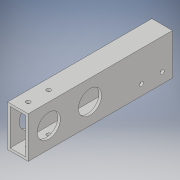
# Autodesk Inventor part: Top Roller Wheel Mount
Saved by Autodesk Inventor 2018 (Build 220112000, 112)
## iProperties
Created: 2020-02-21
Part Number: Top Roller Wheel Mount
Material: Generic
Document SubType Name: Modeling
Designer: T3500STATIC
Density: 1 g/cm^3
Appearance: Default
Author: T3500STATIC
Autodesk Inventor part; units mm, degrees
ref_plane "YZ Plane" through (0, 0, 0) normal (1, 0, 0) x (0, 1, 0)
ref_plane "XZ Plane" through (0, 0, 0) normal (0, 1, 0) x (-1, 0, 0)
ref_plane "XY Plane" through (0, 0, 0) normal (0, 0, 1) x (1, 0, 0)
sketch "Sketch1" plane through (0, 0, 0) normal (1, 0, 0) x (0, 1, 0)
  line L0 (0, 0) -> (50.8, 0)
  line L1 (50.8, 0) -> (50.8, -177.8)
  line L2 (50.8, -177.8) -> (0, -177.8)
  line L3 (0, -177.8) -> (0, 0)
  dimension "d0" = 50.8
  dimension "d1" = 177.8
  constraints: 8 end point, 2 parallel, 1 horizontal, 1 perpendicular
  measures "d0" distance of L1.end L2.end
  measures "d1" distance of L0.end L1.end
extrude "Extrusion1" add sketch "Sketch1" along normal blind 25.4
shell "Shell1" thickness 3.175 removed faces 2 at (8.4667, 16.9333, 0) at (8.4667, 33.8667, -177.8)
sketch "Sketch2" plane through (25.4, 0, 0) normal (1, 0, 0) x (0, 0, -1)
  line L0 (0, 3.175) -> (0, 47.625) construction
  line L1 (0, 25.4) -> (177.8, 25.4) construction
  line L2 (177.8, 3.175) -> (177.8, 47.625) construction
  line L3 (0, 25.4) -> (25.4, 25.4) construction
  circle A0 centre (25.4, 25.4) radius 14.2875
  line L4 (25.4, 25.4) -> (76.2, 25.4) construction
  circle A1 centre (76.2, 25.4) radius 14.2875
  circle A2 centre (25.4, 25.4) radius 19.05 construction
  circle A3 centre (76.2, 25.4) radius 19.05 construction
  line L5 (177.8, 50.8) -> (0, 50.8) construction
  line L6 (0, 50.8) -> (12.7, 50.8) construction
  line L7 (12.7, 50.8) -> (12.7, 38.1) construction
  line L8 (12.7, 38.1) -> (0, 38.1) construction
  line L9 (0, 38.1) -> (0, 50.8) construction
  line L10 (0, 0) -> (12.7, 0) construction
  line L11 (12.7, 0) -> (12.7, 12.7) construction
  line L12 (12.7, 12.7) -> (0, 12.7) construction
  line L13 (0, 12.7) -> (0, 0) construction
  line L14 (177.8, 50.8) -> (165.1, 50.8) construction
  line L15 (165.1, 50.8) -> (165.1, 38.1) construction
  line L16 (165.1, 38.1) -> (177.8, 38.1) construction
  line L17 (177.8, 38.1) -> (177.8, 50.8) construction
  line L18 (177.8, 0) -> (165.1, 0) construction
  line L19 (165.1, 0) -> (165.1, 12.7) construction
  line L20 (165.1, 12.7) -> (177.8, 12.7) construction
  line L21 (177.8, 12.7) -> (177.8, 0) construction
  line L22 (177.8, 50.8) -> (139.7, 50.8) construction
  line L23 (139.7, 50.8) -> (139.7, 38.1) construction
  line L24 (139.7, 38.1) -> (177.8, 38.1) construction
  line L25 (177.8, 38.1) -> (177.8, 50.8) construction
  line L26 (177.8, 0) -> (139.7, 0) construction
  line L27 (139.7, 0) -> (139.7, 12.7) construction
  line L28 (139.7, 12.7) -> (177.8, 12.7) construction
  line L29 (177.8, 12.7) -> (177.8, 0) construction
  circle A4 centre (165.1, 12.7) radius 2.5797
  circle A5 centre (139.7, 12.7) radius 2.5797
  dimension "d5" = 25.4
  dimension "d6" = 28.575
  dimension "d7" = 50.8
  dimension "d8" = 28.575
  dimension "d9" = 38.1
  dimension "d10" = 38.1
  dimension "d11" = 12.7
  dimension "d12" = 12.7
  dimension "d13" = 12.7
  dimension "d14" = 12.7
  dimension "d15" = 12.7
  dimension "d16" = 12.7
  dimension "d17" = 12.7
  dimension "d18" = 12.7
  dimension "d19" = 38.1
  dimension "d20" = 38.1
  dimension "d22" = 5.1594
  dimension "d23" = 5.1594
  constraints: 54 end point, 12 parallel, 6 centre point, 6 coincident, 6 horizontal, 6 perpendicular, 4 point on line, 2 midpoint
  measures "d5" distance of L1.start L3.end
  measures "d6" diameter of A0
  measures "d7" distance of L4.start L4.end
  measures "d8" diameter of A1
  measures "d9" diameter of A2
  measures "d10" diameter of A3
  measures "d11" distance of L7.end L8.end
  measures "d12" distance of L6.end L7.end
  measures "d13" distance of L12.end L11.end
  measures "d14" distance of L11.end L10.end
  measures "d15" distance of L16.end L15.end
  measures "d16" distance of L15.end L14.end
  measures "d17" distance of L19.end L20.end
  measures "d18" distance of L18.end L19.end
  measures "d19" distance of L24.end L23.end
  measures "d20" distance of L27.end L28.end
  measures "d22" diameter of A4
  measures "d23" diameter of A5
extrude "Extrusion2" cut sketch "Sketch2" against normal blind 50.8
hole "Hole1" at (12.7, 0, -12.7) direction (0, 1, 0) diameter 5.1594 end through all
hole "Hole2" at (12.7, 0, -38.1) direction (0, 1, 0) diameter 5.1594 end through all
body "Solid1"
